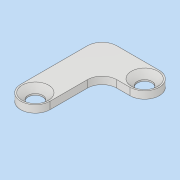
# Autodesk Inventor part: limitSwitchHolder2Backplate
Saved by Autodesk Inventor 2017 (Build 210142000, 142)
## iProperties
Created: 2016-12-17
Part Number: limitSwitchHolder2Backplate
Material: ABS Plastic
Document SubType Name: Modeling
Designer: techn
Density: 1.06 g/cm^3
Appearance: Smooth - White
Author: techn
Autodesk Inventor part; units mm, degrees
ref_plane "YZ Plane" through (0, 0, 0) normal (1, 0, 0) x (0, 1, 0)
ref_plane "XZ Plane" through (0, 0, 0) normal (0, 1, 0) x (-1, 0, 0)
ref_plane "XY Plane" through (0, 0, 0) normal (0, 0, 1) x (1, 0, 0)
sketch "Sketch1" plane through (0, 0, 0) normal (0, 1, 0) x (-1, 0, 0)
  circle A0 centre (0, 0) radius 1.5875
  line L0 (3.175, 3.175) -> (-3.175, 3.175)
  line L1 (-3.175, 3.175) -> (-3.175, -15.24)
  line L2 (-3.175, -15.24) -> (3.175, -15.24)
  line L3 (3.175, -15.24) -> (3.175, 3.175)
  dimension "d0" = 3.175
  dimension "d1" = 3.175
  dimension "d2" = 3.175
  dimension "d3" = 3.175
  dimension "d4" = 15.24
  constraints: 8 end point, 2 parallel, 1 centre point, 1 coincident, 1 horizontal, 1 perpendicular
  measures "d0" diameter of A0
  measures "d1" distance from line of L3 point (0, 0)
  measures "d2" distance from line of L1 point (0, 0)
  measures "d3" distance from line of point (0, 0) L0
  measures "d4" distance from line of L2 point (0, 0)
extrude "Extrusion1" add sketch "Sketch1" along normal blind 1.5875
chamfer "Chamfer1" distance 1.27 angle 45 1 edges at (1.5875, 1.5875, 0)
sketch "Sketch2" plane through (0, 1.5875, 0) normal (0, 1, 0) x (1, 0, 0)
  line L0 (-3.175, 15.24) -> (-3.175, -3.175) projected
  line L1 (3.175, -3.175) -> (3.175, 15.24) projected
  circle A0 centre (0, 0) radius 2.8575 projected
  circle A1 centre (9.2075, 14.4379) radius 1.5875
  circle A2 centre (9.2075, 14.4379) radius 3.175
  line L2 (9.2075, 17.6129) -> (3.175, 17.6129)
  line L3 (3.175, 0) -> (3.175, 15.875) projected
  line L4 (9.2075, 11.2629) -> (3.175, 11.2629)
  line L5 (-3.175, -3.175) -> (3.175, -3.175) projected
  line L6 (3.175, 15.24) -> (-3.175, 15.24) projected
  line L7 (3.175, 17.6129) -> (-3.175, 17.6129)
  line L8 (3.175, 15.24) -> (-3.175, 15.24) projected
  line L9 (-3.175, 17.6129) -> (-3.175, 15.24)
  line L10 (3.175, -3.175) -> (3.175, 15.24) projected
  line L11 (-3.175, 15.24) -> (3.175, 15.24)
  line L12 (3.175, 15.24) -> (3.175, 11.2629)
  dimension "d11" = 9.2075
  dimension "d12" = 14.4379
  dimension "d13" = 3.175
  dimension "d14" = 6.35
  constraints: 12 end point, 4 perpendicular, 2 centre point, 2 horizontal, 2 point on circle, 2 point on line, 1 coincident, 1 tangent
  measures "d11" horizontal distance of point (0, 0) A1.centre
  measures "d12" vertical distance of point (0, 0) A1.centre
  measures "d13" diameter of A1
  measures "d14" diameter of A2
extrude "Extrusion3" add sketch "Sketch2" against normal up to surface (1.5875 mm away) contours L9 L7 L2 A2 L4 L1 L6 | A2
fillet "Fillet3" radius 3.175 4 edges at (3.175, 0.7937, -11.2629) (-3.175, 0.7937, -17.6129) (-3.175, 0.7937, 3.175) (3.175, 0.7937, 3.175)
chamfer "Chamfer3" distance 1.27 angle 45 1 edges at (7.62, 1.5875, -14.4379)
body "Solid1"
